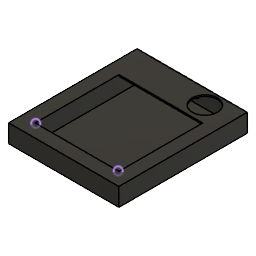
MACROPAD V3 (Autodesk Fusion 360 design; units mm, degrees)
part number: 2026-03-01-07-29-17-711
Autodesk Fusion 360 part; units mm, degrees
note: some values were not read from the file. Chosen so that the rebuilt part matches the saved one: which face or edge a step refers to; that a step has no effect; which pieces of a blend or face edit are solid.
sketch "Sketch1" plane through (0, 0, 0) normal (0, 1, 0) x (1, 0, 0)
  line L0 (10.4015, -9.958) -> (69.4515, -9.958)
  line L1 (69.4515, -9.958) -> (69.4515, -92.483)
  line L2 (69.4515, -92.483) -> (10.4015, -92.483)
  line L3 (10.4015, -92.483) -> (10.4015, -9.958)
  line L4 (0.3153, 0.0894) -> (79.3653, 0.0894)
  line L5 (79.3653, 0.0894) -> (79.3653, -101.9106)
  line L6 (79.3653, -101.9106) -> (0.3153, -101.9106)
  line L7 (0.3153, -101.9106) -> (0.3153, 0.0894)
  dimension "d1" = 59.05
  dimension "d2" = 82.525
  dimension "d3" = 102
  dimension "d4" = 79.05
  constraint horizontal L0
  constraint vertical L1
  constraint horizontal L2
  constraint vertical L3
  constraint horizontal L4
  constraint vertical L5
  constraint horizontal L6
  constraint vertical L7
  measures "d1" distance of L0.start L0.end
  measures "d2" distance of L0.start L2.end
  measures "d3" distance of L4.end L5.end
  measures "d4" distance of L5.end L6.end
extrude "Extrude1" add sketch "Sketch1" along normal blind 13 makes body 1
sketch "Sketch2" plane through (0, 0, 0) normal (0, 1, 0) x (1, 0, 0)
  line L0 (10, -10) -> (70, -10)
  line L1 (70, -10) -> (70, -93)
  line L2 (70, -93) -> (10, -93)
  line L3 (10, -93) -> (10, -10)
  constraint horizontal L0
  constraint vertical L1
  constraint horizontal L2
  constraint vertical L3
extrude "Extrude2" add sketch "Sketch2" along normal blind 1 bodies 1
sketch "Sketch3" plane through (0, 0, 0) normal (0, 1, 0) x (1, 0, 0)
  line L0 (115, -10) -> (175.01, -10)
  line L1 (175.01, -10) -> (175.01, -32.475)
  line L2 (175.01, -32.475) -> (115, -32.475)
  line L3 (115, -32.475) -> (115, -10)
  dimension "d11" = 22.475
  dimension "d12" = 60.01
  constraint horizontal L0
  constraint vertical L1
  constraint horizontal L2
  constraint vertical L3
  measures "d11" distance of L0.start L2.end
  measures "d12" distance of L0.start L0.end
extrude "Extrude3" add sketch "Sketch3" along normal blind 1 separate body makes body 2
move_body "Move1" bodies 2 to x (1, 0, 0) y (0, 1, 0) z (0, 0, 1) at (0, 14, 0)
move_body "Move2" bodies 2 to x (1, 0, 0) y (0, 1, 0) z (0, 0, 1) at (-105, 0, 0)
sketch "Sketch4" plane through (0, 13, 0) normal (0, 1, 0) x (-1, 0, 0)
  line L0 (-69.4515, 92.483) -> (-10.4015, 92.483)
hole "Hole1" at (59.6437, 15, 20.5599) direction (0, -1, 0) diameter 18 depth 12 tip angle 180 bodies 2
delete_face "DeleteFace1" [no effect]
move_face "MoveFace1" by (38, 0, 0) 1 faces at (23.5563, 15, 21.2358) on bodies 2
move_body "Move3" bodies 2 to x (1, 0, 0) y (0, 1, 0) z (0, 0, 1) at (0, -2, 0)
move_face "MoveFace2" by (0, 0, 10) 1 faces at (26.6653, 4.3333, -0.0894) on bodies 1
move_face "MoveFace3" by (-1, 0, 0) 1 faces at (26.6653, 4.3333, 9.9106) on bodies 1
move_face "MoveFace4" by (-1, 0, 0) 1 faces at (10.4015, 9, 37.4803) on bodies 1
move_face "MoveFace5" by (0.6, 0, 0) 1 faces at (9.4015, 9, 37.4803) on bodies 1
move_face "MoveFace6" by (0.4, 0, 0) 1 faces at (69.4515, 9, 37.4803) on bodies 1
move_face "MoveFace7" by (0.15, 0, 0) 1 faces at (69.8515, 9, 37.4803) on bodies 1
sketch "Sketch5" plane through (0, 0, 0) normal (0, 1, 0) x (1, 0, 0)
  line L0 (37.8086, -7.5268, 3.7627) -> (46.2086, -7.5332, 3.7627)
  arc A0 through (46.2086, -7.5332, 3.7627) (48.8086, -7.5351, 6.3627) (46.2086, -7.5332, 8.9627)
  line L1 (46.2086, -7.5332, 8.9627) -> (37.8086, -7.5268, 8.9627)
  arc A1 through (37.8086, -7.5268, 8.9627) (35.2086, -7.5248, 6.3627) (37.8086, -7.5268, 3.7627)
  line L2 (35.2086, -7.5248, 6.3627) -> (48.8086, -7.5351, 6.3627) construction
  dimension "d20" = 8.4
  dimension "d21" = 2.6
sketch "Sketch5 (curves on the plane with normal 0.0008, 0, -1 at -7.4982 mm)" plane through (-0.0057, 0, 7.4982) normal (0.000758, 0, -1) x (-1, 0, -0.000758)
  line L0 (-37.8143, 3.7627) -> (-46.2143, 3.7627)
  arc A0 (-46.2143, 3.7627) -> (-46.2143, 8.9627) centre (-46.2143, 6.3627) cw
  line L1 (-46.2143, 8.9627) -> (-37.8143, 8.9627)
  arc A1 (-37.8143, 8.9627) -> (-37.8143, 3.7627) centre (-37.8143, 6.3627) cw
  line L2 (-35.2143, 6.3627) -> (-48.8143, 6.3627) construction
extrude "Extrude4" cut sketch "Sketch5 (curves on the plane with normal 0.0008, 0, -1 at -7.4982 mm)" against normal blind 35 bodies 1
move_face "MoveFace8" by (0, 18, 0) 1 faces at (11.9458, 6.4542, 9.9106) on bodies 1
move_face "MoveFace9" by (34, 0, 0) 1 faces at (11.9458, 6.4542, 9.9106) on bodies 1
sketch "Sketch6" plane through (0, 0, 0) normal (0, 0, 1) x (1, 0, 0)
  line L0 (52, 11) -> (32, 11)
  line L1 (32, 11) -> (32, 3)
  line L2 (32, 3) -> (52, 3)
  line L3 (52, 3) -> (52, 11)
  constraint horizontal L0
  constraint vertical L1
  constraint horizontal L2
  constraint vertical L3
extrude "Extrude5" add sketch "Sketch6" against normal blind 1 separate body makes body 3
move_body "Move4" bodies 3 to x (1, 0, 0) y (0, 1, 0) z (0, 0, 1) at (0, 0, 13)
move_face "MoveFace10" by (0, 0, -1) 1 faces at (38.6667, 8.3333, 12) on bodies 3
move_face "MoveFace11" by (0, 0, -1) 1 faces at (38.6667, 8.3333, 11) on bodies 3
extrude "Extrude6" add 1 faces at (11.9458, 6.4542, 9.9106) along direction (0, 0, -1) blind 0.07 on bodies 1 bodies 1
move_face "MoveFace12" by (-63, 0, 0) 1 faces at (11.9458, 6.4542, 9.8406) on bodies 1
delete_face "DeleteFace2" 1 faces at (18.4032, 6.4542, 9.958) on bodies 1
move_body "Move5" bodies 3 to x (1, 0, 0) y (0, 1, 0) z (0, 0, 1) at (-2.5143, 29.0863, 0.9686)
extrude "Extrude7" cut 1 faces at (36.1523, 37.4196, 10.9686) along direction (0, 0, 1) blind 2 on bodies 3 bodies 3
move_body "Move6" bodies 3 to x (1, 0, 0) y (0, 1, 0) z (0, 0, 1) at (29, -28, -3.2)
extrude "Extrude8" add 1 faces at (58.4857, 9.4196, 10.4352) along direction (-1, 0, 0) blind 58.17 on bodies 3 bodies 1 3 2
extrude "Extrude9" add 1 faces at (78.4857, 9.4196, 9.7926) along direction (1, 0, 0) blind 0.83 on bodies 1 bodies 1
extrude "Extrude10" add 1 faces at (50.0015, 12.0863, 9.9469) along direction (0, 1, 0) blind 0.914 on bodies 1 bodies 1
extrude "Extrude11" cut 1 faces at (50.0015, 4.0863, 10.1499) along direction (0, -1, 0) blind 4.1 on bodies 1 bodies 1
extrude "Extrude12" add 1 faces at (50.0015, 4.0863, 10.1499) along direction (0, -1, 0) blind 4.1 on bodies 1 bodies 1
sketch "Sketch7" plane through (0, 0, 0) normal (0, 0, 1) x (1, 0, 0)
  line L0 (42.6529, 10.8769, 3) -> (33.6529, 10.8769, 3)
  arc A0 through (33.6529, 10.8769, 3) (30.1529, 7.3769, 3) (33.6529, 3.8769, 3)
  line L1 (33.6529, 3.8769, 3) -> (42.6529, 3.8769, 3)
  arc A1 through (42.6529, 3.8769, 3) (46.1529, 7.3769, 3) (42.6529, 10.8769, 3)
  line L2 (46.1529, 7.3769, 3) -> (30.1529, 7.3769, 3) construction
  dimension "d40" = 9
  dimension "d41" = 3.5
sketch "Sketch7 (curves 3 mm off its plane)" plane through (0, 0, 3) normal (0, 0, 1) x (1, 0, 0)
  line L0 (42.6529, 10.8769) -> (33.6529, 10.8769)
  arc A0 (33.6529, 10.8769) -> (33.6529, 3.8769) centre (33.6529, 7.3769) ccw
  line L1 (33.6529, 3.8769) -> (42.6529, 3.8769)
  arc A1 (42.6529, 3.8769) -> (42.6529, 10.8769) centre (42.6529, 7.3769) ccw
  line L2 (46.1529, 7.3769) -> (30.1529, 7.3769) construction
extrude "Extrude13" cut sketch "Sketch7 (curves 3 mm off its plane)" along normal blind 18 bodies 1
